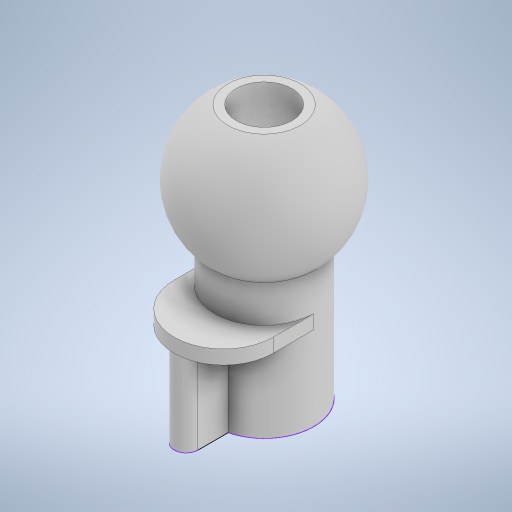
# Autodesk Inventor part: New_11_Base_Joint
Saved by Autodesk Inventor 2024.2 (Build 282272000, 272)
## iProperties
Created: 2025-05-26
Part Number: New_11_Base_Joint
Material: Všeobecné
Document SubType Name: Modeling
Designer: Elite
Density: 1 g/cm^3
Appearance: Výchozí
Author: Elite
Autodesk Inventor part; units mm, degrees
ref_plane "YZ Plane" through (0, 0, 0) normal (1, 0, 0) x (0, 1, 0)
ref_plane "XY Plane" through (0, 0, 0) normal (0, 0, 1) x (1, 0, 0)
sketch "Náčrt2" plane through (0, 0, 0) normal (1, 0, 0) x (0, 1, 0)
  line L0 (-2.5936, 18.2) -> (2.6216, 18.2) projected
  line L1 (-6.458, 6.9989) -> (0.6548, 6.9989) projected
  line L2 (-3.5412, 9.6623) -> (3.7182, 9.6623) projected
  line L3 (0, 18.2) -> (0, 9.6623)
  arc A0 (-2.5936, 18.2) -> (-3.5412, 9.6623) centre (0.0066, 13.59) ccw
  line L4 (0, 18.2) -> (0, 0)
  constraints: 4 end point, 2 point on circle, 2 point on line, 1 centre point, 1 perpendicular, 1 vertical
revolve "Rotace1" add sketch "Náčrt2" angle 360 about axis through (0, 0, 18.2) along (0, 0, -1)
sketch "Náčrt3" plane through (0, 0, 18.2) normal (0, 0, 1) x (1, 0, 0)
  circle A0 centre (0, 0) radius 2
  dimension "d1" = 4
  constraints: 1 centre point, 1 coincident
  measures "d1" diameter of A0
extrude "Vysunutí1" cut sketch "Náčrt3" against normal blind 10
sketch "Náčrt4" plane through (-3.5364, -0.0875, 0) normal (0, 0, -1) x (-1, 0, 0)
  circle A0 centre (-3.5364, 0.0875) radius 3.5412 projected
  circle A1 centre (-3.5364, 0.0875) radius 2 projected
  line L0 (-2.6864, -5.5125) -> (-2.6864, -3.3464) projected
  circle A2 centre (-3.5364, -5.5125) radius 0.85 projected
  line L1 (-4.3864, -3.3464) -> (-4.3864, -5.5125) projected
  point P0 (-3.5364, 0.0875)
  point P1 (-4.3864, -3.3502)
  point P2 (-2.6864, -3.3502)
extrude "Vysunutí2" add sketch "Náčrt4" against normal blind 10 contours A0
sketch "Náčrt5" plane through (-3.5364, -0.0875, 0) normal (0, 0, -1) x (-1, 0, 0)
  point P0 (-3.5364, 0.0875)
extrude "Vysunutí3" add sketch "Náčrt4" against normal blind 7 contours A0 L0 A2 L1 | A2
sketch "Náčrt6" plane through (0, 0, 0) normal (0, 1, 0) x (-1, 0, 0)
  line L0 (0, 0) -> (-1.2, 0)
  line L1 (2, 0) -> (-2, 0) projected
  line L2 (-1.2, 0) -> (-1.2, 7.5)
  line L3 (-1.2, 7.5) -> (1.2, 7.5)
  line L4 (1.2, 7.5) -> (1.2, 0)
  arc A0 (1.2, 7.5) -> (-1.2, 7.5) centre (0, 7.5) ccw
  line L5 (0, 0) -> (1.2, 0)
  line L6 (-1.2, 7.5) -> (1.2, 7.5)
  line L7 (-1.2, 0) -> (1.2, 0)
  line L8 (1.2, 7.5) -> (1.2, 0)
  line L9 (1.2, 7.5) -> (-1.2, 7.5)
  line L10 (-1.2, 7.5) -> (-1.2, 0)
  dimension "d11" = 1.2
  dimension "d12" = 7.5
  dimension "d13" = 2.4
  constraints: 20 end point, 4 collinear, 4 perpendicular, 2 point on circle, 2 point on line, 2 tangent, 1 centre point, 1 parallel
  measures "d11" distance of L0.start L0.end
  measures "d12" distance of L0.end L2.end
  measures "d13" distance of L2.end L3.end
ref_plane "Pracovní rovina1" through (0, 2.75, 0) normal (0, 1, 0) x (-1, 0, 0)
sketch "Náčrt7" plane through (0, 0, 0) normal (0, 1, 0) x (-1, 0, 0)
  line L0 (1.2, 7.447) -> (1.2, 0) projected
  line L1 (-1.2, 7.447) -> (1.2041, 7.447)
  line L2 (1.2041, 7.447) -> (1.2041, 7.4445)
  line L3 (-1.2, 7.4445) -> (-1.2, 7.447)
  line L4 (1.2, 7.4445) -> (1.2, 0)
  line L5 (1.2, 0) -> (-1.2, 0)
  ellipse E0 centre (0.0021, 7.4458) end of major axis (0.0038, 9.0631) minor radius 1.2021 (1.2041, 7.4445) -> (-1.2, 7.4355) ccw
  line L6 (1.2, 7.4445) -> (1.2, 7.447)
  line L7 (1.2, 7.447) -> (-1.2, 7.447)
  line L8 (-1.2, 7.447) -> (-1.2, 7.4445)
  line L9 (-1.2, 0) -> (1.2041, 0)
  line L10 (1.2041, 0) -> (1.2041, 7.447)
  line L11 (1.2041, 7.447) -> (-1.2, 7.447)
  line L12 (-1.2, 7.447) -> (-1.2, 0)
  point P0 (0, 0)
  dimension "d9" = 2.4
  dimension "d10" = 7.447
  constraints: 24 end point, 4 parallel, 2 horizontal, 2 perpendicular, 4 other
  measures "d9" distance of L0.end L5.end
  measures "d10" distance of L11.end L5.end
extrude "Vysunutí4" cut sketch "Náčrt6" along normal blind 10
sketch "Náčrt8" plane through (-3.5364, -0.0875, 7) normal (0, 0, 1) x (1, 0, 0)
  arc A0 (2.6864, -5.5125) -> (4.3864, -5.5125) centre (3.5364, -5.5125) ccw projected
  line L0 (2.6864, -3.3502) -> (2.6864, -5.5125) projected
  line L1 (4.3864, -5.5125) -> (4.3864, -3.3502) projected
  arc A1 (4.3864, -3.3502) -> (2.6864, -3.3502) centre (3.5364, 0.0875) ccw projected
  arc A2 (4.3864, -3.3502) -> (4.7364, 3.4192) centre (3.5364, 0.0875) ccw projected
  arc A3 (2.3364, 1.6875) -> (4.7364, 1.6875) centre (3.5364, 0.0875) ccw projected
  circle A4 centre (3.5422, -2.8248) radius 3.5391 projected
  line L2 (4.3864, -3.3502) -> (4.3864, -5.5125) projected
  arc A5 (2.6864, -5.5125) -> (4.3864, -5.5125) centre (3.5364, -5.5125) ccw projected
  line L3 (2.6864, -5.5125) -> (2.6864, -3.3502) projected
  line L4 (7.0813, -2.8203) -> (7.0776, 0.092)
  line L5 (0.003, -2.8342) -> (-0.0048, 0.078)
  line L6 (2.6864, -5.5125) -> (2.6864, -3.3502) projected
  arc A6 (2.6864, -5.5125) -> (4.3864, -5.5125) centre (3.5364, -5.5125) ccw projected
  arc A7 (2.3364, 3.4192) -> (2.6864, -3.3502) centre (3.5364, 0.0875) ccw projected
  line L7 (4.3864, -3.3502) -> (4.3864, -5.5125) projected
  arc A8 (2.6864, -5.5125) -> (4.3864, -5.5125) centre (3.5364, -5.5125) ccw projected
  line L8 (2.6864, -5.5125) -> (2.6864, -3.3502) projected
  arc A9 (2.3364, 1.6875) -> (4.7364, 1.6875) centre (3.5364, 0.0875) ccw projected
  line L9 (4.7364, 1.6875) -> (4.7364, 3.4192) projected
  arc A10 (4.3864, -3.3502) -> (4.7364, 3.4192) centre (3.5364, 0.0875) ccw projected
  line L10 (2.3364, 3.4192) -> (2.3364, 1.6875) projected
  line L11 (4.7364, 1.6875) -> (4.7364, 3.4192) projected
  arc A11 (2.3364, 3.4192) -> (2.6864, -3.3502) centre (3.5364, 0.0875) ccw projected
  line L12 (2.3364, 3.4192) -> (2.3364, 1.6875) projected
  point P0 (3.5364, 0.0875)
  point P1 (7.0776, 0.092)
  point P2 (-0.0048, 0.078)
  constraints: 4 end point, 4 point on circle, 4 tangent
extrude "Vysunutí5" add sketch "Náčrt8" against normal blind 1 contours A0 A4 A1 L0 | A0 L1 A1 A4 | L5 A1 A4 | A4 A1 L4
sketch "Náčrt9" plane through (-3.5364, -0.0875, 0) normal (0, 0, -1) x (-1, 0, 0)
  circle A0 centre (-3.5364, 0.0875) radius 2
  circle A1 centre (-3.5364, 0.0875) radius 3.5412
  circle A2 centre (-3.5364, -5.5125) radius 0.85
  line L0 (-4.3864, -5.5125) -> (-4.3864, -3.3502)
  line L1 (-2.6864, -5.5125) -> (-2.6864, -3.3502)
  line L2 (-4.7364, 1.6875) -> (-4.7364, 3.4192)
  line L3 (-2.3364, 1.6875) -> (-2.3364, 3.4192)
  point P0 (-3.5364, 0.0875)
  constraints: 8 end point, 3 centre point, 3 coincident, 2 parallel, 1 vertical
